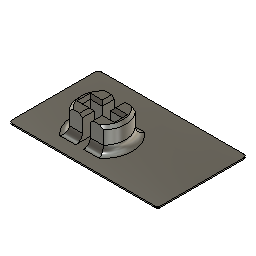
iNTEX_1.75u_Stepped (Autodesk Fusion 360 design; units mm, degrees)
Autodesk Fusion 360 part; units mm, degrees
sketch "Sketch1" plane through (0, 0, 0) normal (0, 0, 1) x (1, 0, 0)
  line L0 (16.3, 9) -> (-16.3, 9) construction
  line L1 (-16.3, 9) -> (-16.3, -9) construction
  line L2 (-16.3, -9) -> (16.3, -9) construction
  line L3 (16.3, -9) -> (16.3, 9) construction
  line L4 (16.3, 9) -> (-16.3, -9) construction
  line L5 (-16.3, 9) -> (16.3, -9) construction
  line L6 (-8.6, 8) -> (13.7, 8)
  line L7 (13.7, 8) -> (13.7, -5.4)
  line L8 (13.7, -5.4) -> (-8.6, -5.4)
  line L9 (-8.6, -5.4) -> (-8.6, 8)
  circle A0 centre (0, 0) radius 3.5
  line L10 (2.4, -0.6) -> (-2.4, -0.6)
  line L11 (-2.4, -0.6) -> (-2.4, 0.6)
  line L12 (-2.4, 0.6) -> (2.4, 0.6)
  line L13 (2.4, 0.6) -> (2.4, -0.6)
  line L14 (2.4, -0.6) -> (-2.4, 0.6) construction
  line L15 (-2.4, -0.6) -> (2.4, 0.6) construction
  line L16 (0.6, -2.4) -> (-0.6, -2.4)
  line L17 (-0.6, -2.4) -> (-0.6, 2.4)
  line L18 (-0.6, 2.4) -> (0.6, 2.4)
  line L19 (0.6, 2.4) -> (0.6, -2.4)
  line L20 (0.6, -2.4) -> (-0.6, 2.4) construction
  line L21 (-0.6, -2.4) -> (0.6, 2.4) construction
  line L22 (-0.6, 2.4) -> (-2.5475, 2.4)
  line L23 (0.6, 2.4) -> (2.5475, 2.4)
  line L24 (-0.6, -2.4) -> (-2.5475, -2.4)
  line L25 (0.6, -2.4) -> (2.5475, -2.4)
  dimension "d1" = 32.6
  dimension "d2" = 18
  dimension "d3" = 3.6
  dimension "d4" = 1
  dimension "d5" = 2.6
  dimension "d6" = 7.7
  dimension "d7" = 7
  dimension "d8" = 4.8
  dimension "d9" = 1.2
  dimension "d10" = 1.2
  dimension "d11" = 4.8
  constraint perpendicular L0 L1
  constraint parallel L0 L2
  constraint parallel L1 L3
  constraint horizontal L0
  constraint coincident L4 A0.centre
  constraint coincident L5 A0.centre
  constraint coincident A0.centre origin
  constraint horizontal L6
  constraint vertical L7
  constraint horizontal L8
  constraint vertical L9
  constraint perpendicular L10 L11
  constraint parallel L10 L12
  constraint parallel L11 L13
  constraint horizontal L10
  constraint coincident L14 A0.centre
  constraint coincident L15 A0.centre
  constraint perpendicular L16 L17
  constraint parallel L16 L18
  constraint parallel L17 L19
  constraint horizontal L16
  constraint coincident L20 A0.centre
  constraint coincident L21 A0.centre
  constraint coincident A0 L22.end
  constraint perpendicular L17 L22
  constraint coincident A0 L23.end
  constraint perpendicular L19 L23
  constraint coincident A0 L24.end
  constraint perpendicular L17 L24
  constraint coincident A0 L25.end
  constraint perpendicular L19 L25
  measures "d1" distance of L1.end L2.end
  measures "d2" distance of L0.end L1.end
  measures "d4" distance of L0 L6
  measures "d5" distance of L3 L7
  measures "d6" distance of L1 L9
  measures "d7" diameter of A0
  measures "d8" distance of L11.end L12.end
  measures "d9" distance of L10.end L11.end
  measures "d10" distance of L17.end L18.end
  measures "d11" distance of L16.end L17.end
extrude "Extrude1" add sketch "Sketch1" along normal blind 0.6 contours L6 L7 L8 L9 | A0 L10 L12 L13 L19 L23 L25 | A0 L18 L22 L23 | A0 L16 L24 L25 | A0 L10 L11 L12 L17 L22 L24 | L12 L17 L18 L19 | L10 L16 L17 L19 | L10 L12 L17 L19 | L10 L12 L13 L19 | L10 L11 L12 L17
extrude "Extrude2" add sketch "Sketch1" along normal blind 4 contours A0 L10 L12 L13 L19 L23 L25 | A0 L10 L11 L12 L17 L22 L24
fillet "Fillet1" radius 1 6 edges at (-1.5738, -2.4, 0.6) (-3.5, 0, 0.6) (1.5738, -2.4, 0.6) (3.5, 0, 0.6) (1.5738, 2.4, 0.6) (-1.5738, 2.4, 0.6)
fillet "Fillet1" radius 0.5 4 edges at (13.7, 8, 0.3) (-8.6, 8, 0.3) (13.7, -5.4, 0.3) (-8.6, -5.4, 0.3)
chamfer "Chamfer1" distance 0.4 angle 45 20 edges at (-8.4536, 7.8536, 0) (2.55, 8, 0) (13.5536, 7.8536, 0) (13.7, 1.3, 0) (13.5536, -5.2536, 0) (2.55, -5.4, 0) (-8.4536, -5.2536, 0) (-8.6, 1.3, 0) (-0.6, 1.5, 4) (-1.5, 0.6, 4) (-2.4, 0, 4) (-1.5, -0.6, 4) (-0.6, -1.5, 4) (0.6, -1.5, 4) (1.5, -0.6, 4) (2.4, 0, 4) (1.5, 0.6, 4) (0.6, 1.5, 4) (3.5, 0, 4) (-3.5, 0, 4)
named bodies: "iNTEX_1.75u_Stepped"
